Autodesk Inventor part; units mm, degrees
(part 2 of 2)
sketch "スケッチ16" plane through (0, 0, 3) normal (0, 0, 1) x (1, 0, 0)
  line L0 (-24.4121, 84.9889) -> (-12.8854, 81.652) projected
  arc A0 (-12.8854, 81.652) -> (-13.4416, 79.7309) centre (-13.1635, 80.6914) ccw projected
  line L1 (-13.4416, 79.7309) -> (-16.2223, 70.1253) projected
  arc A1 (-16.2223, 70.1253) -> (-16.7785, 68.2042) centre (-16.5004, 69.1647) ccw projected
  line L2 (-16.7785, 68.2042) -> (-28.3052, 71.5411) projected
  arc A2 (-28.3052, 71.5411) -> (-27.749, 73.4622) centre (-28.0271, 72.5017) ccw projected
  line L3 (-27.749, 73.4622) -> (-24.9683, 83.0678) projected
  arc A3 (-24.9683, 83.0678) -> (-24.4121, 84.9889) centre (-24.6902, 84.0284) ccw projected
  circle A4 centre (-11.9503, 74.0939) radius 1.5 projected
  circle A5 centre (-6.1515, 120.3493) radius 1.5 projected
  circle A6 centre (-24.1421, 119.7668) radius 1.5 projected
  circle A7 centre (-29.2403, 79.0993) radius 1.5 projected
  arc A8 (-9.3765, 127.2485) -> (-9.3118, 125.2496) centre (-9.3441, 126.249) ccw projected
  line L4 (-9.3118, 125.2496) -> (-8.9882, 115.2548) projected
  arc A9 (-8.9882, 115.2548) -> (-8.9234, 113.2558) centre (-8.9558, 114.2553) ccw projected
  line L5 (-8.9234, 113.2558) -> (-20.9172, 112.8675) projected
  arc A10 (-20.9172, 112.8675) -> (-20.9819, 114.8665) centre (-20.9495, 113.867) ccw projected
  line L6 (-20.9819, 114.8665) -> (-21.3055, 124.8612) projected
  arc A11 (-21.3055, 124.8612) -> (-21.3702, 126.8602) centre (-21.3378, 125.8607) ccw projected
  line L7 (-21.3702, 126.8602) -> (-9.3765, 127.2485) projected
  circle A12 centre (55.4, 111) radius 1.25 projected
  circle A13 centre (25, 100.25) radius 1.5 projected
  circle A14 centre (0, 66.75) radius 1.5 projected
  circle A15 centre (25, 66.75) radius 1.5 projected
  circle A16 centre (0, 100.25) radius 1.5 projected
  circle A17 centre (55.3, 64) radius 1.6 projected
  line L8 (23, 137) -> (23, 140) projected
  arc A18 (23, 140) -> (25, 140) centre (24, 140) ccw projected
  line L9 (25, 140) -> (29, 140) projected
  arc A19 (29, 140) -> (29.866, 138.5) centre (29, 139) ccw projected
  arc A20 (29.866, 138.5) -> (29, 137) centre (29, 138) ccw projected
  line L10 (29, 137) -> (25, 137) projected
  arc A21 (25, 137) -> (23, 137) centre (24, 137) ccw projected
  line L11 (51, 140) -> (55, 140) projected
  arc A22 (55, 140) -> (57, 140) centre (56, 140) ccw projected
  line L12 (57, 140) -> (57, 137) projected
  arc A23 (57, 137) -> (55, 137) centre (56, 137) ccw projected
  line L13 (55, 137) -> (51, 137) projected
  arc A24 (51, 137) -> (50.134, 138.5) centre (51, 138) ccw projected
  arc A25 (50.134, 138.5) -> (51, 140) centre (51, 139) ccw projected
  line L14 (37, 137) -> (37, 140) projected
  arc A26 (37, 140) -> (39, 140) centre (38, 140) ccw projected
  line L15 (39, 140) -> (43, 140) projected
  arc A27 (43, 140) -> (43.866, 138.5) centre (43, 139) ccw projected
  arc A28 (43.866, 138.5) -> (43, 137) centre (43, 138) ccw projected
  line L16 (43, 137) -> (39, 137) projected
  arc A29 (39, 137) -> (37, 137) centre (38, 137) ccw projected
  circle A30 centre (-12.461, 47.5151) radius 1.2295 projected
  circle A31 centre (-34.1345, 137.9496) radius 1.2295 projected
  circle A32 centre (-19.3858, 140.684) radius 1.2295 projected
  circle A33 centre (-30.5132, 56.1243) radius 1.2295 projected
  circle A34 centre (-1.5, 36) radius 1.6 projected
  circle A35 centre (-1.5, 144) radius 1.6 projected
  circle A36 centre (30, 16) radius 1.6 projected
  circle A37 centre (30, 124) radius 1.6 projected
  line L17 (62.5, 150) -> (-47.5, 150) projected
  line L18 (-47.5, 150) -> (-47.5, 10) projected
  line L19 (-47.5, 10) -> (62.5, 10) projected
  line L20 (62.5, 10) -> (62.5, 150) projected
  arc A38 (59.9998, 139.9632) -> (56.3191, 143.9873) centre (56, 140) ccw
  arc A39 (-35.0095, 55.9402) -> (-33.9034, 53.1651) centre (-30.5132, 56.1243) ccw
  arc A40 (-34.9519, 142.0993) -> (-38.3604, 137.7765) centre (-34.1345, 137.9496) ccw
  line L21 (-20.2327, 144.9986) -> (-34.9519, 142.0993)
  line L22 (-38.3604, 137.7765) -> (-35.0095, 55.9402)
  line L23 (6.5, 10) -> (30, 10)
  line L24 (59.2998, 63.9632) -> (59.9998, 139.9632)
  arc A41 (-1.133, 148.5853) -> (-2.389, 148.5133) centre (-1.5, 144) ccw
  line L25 (-20.2327, 144.9986) -> (-2.389, 148.5133)
  line L26 (-1.133, 148.5853) -> (56.3191, 143.9873)
  circle A42 centre (21.5, 22) radius 1.6 projected
  arc A43 (18.5, 15) -> (18.5, 17) centre (18.5, 16) ccw projected
  line L27 (18.5, 15) -> (6.5, 15) projected
  arc A44 (6.5, 17) -> (6.5, 15) centre (6.5, 16) ccw projected
  line L28 (6.5, 17) -> (6.5, 27) projected
  arc A45 (6.5, 29) -> (6.5, 27) centre (6.5, 28) ccw projected
  line L29 (6.5, 29) -> (18.5, 29) projected
  arc A46 (18.5, 27) -> (18.5, 29) centre (18.5, 28) ccw projected
  line L30 (18.5, 27) -> (18.5, 17) projected
  circle A47 centre (3.5, 22) radius 1.6 projected
  arc A48 (1.9797, 12.0545) -> (6.5, 10) centre (6.5, 16) ccw
  line L31 (-33.9034, 53.1651) -> (1.9797, 12.0545)
  circle A49 centre (43.2987, 57.3213) radius 1.25 projected
  circle A50 centre (43.3013, 22.6802) radius 1.25 projected
  line L32 (35.3, 23.7) -> (33.3, 23.7) projected
  line L33 (33.3, 56.3) -> (35.3, 56.3) projected
  circle A51 centre (13.3, 39.9985) radius 1.25 projected
  circle A52 centre (55.4, 87) radius 1.2295 projected
  arc A53 (45.0562, 20.5259) -> (42.136, 25.2027) centre (43.3013, 22.6802) ccw
  arc A54 (30, 10) -> (33.7894, 11.3481) centre (30, 16) ccw
  line L34 (33.7894, 11.3481) -> (45.0562, 20.5259)
  arc A55 (56.9267, 60.3457) -> (59.2998, 63.9632) centre (55.3, 64) ccw
  arc A56 (42.1337, 54.7983) -> (44.4288, 54.7825) centre (43.2987, 57.3213) ccw
  line L35 (56.9267, 60.3457) -> (44.4288, 54.7825)
  arc A57 (35.3, 23.7) -> (42.136, 25.2027) centre (35.3, 40) ccw
  arc A58 (42.1337, 54.7983) -> (35.3, 56.3) centre (35.3, 40) ccw
  arc A59 (33.3, 56.3) -> (33.3, 23.7) centre (33.3, 40) ccw
  point P0 (0, 0)
  dimension "d161" = 3
  dimension "d163" = 3
  dimension "d164" = 4
  dimension "d185" = 6
  dimension "d206" = 4
  dimension "d207" = 6
  dimension "d209" = 12
  dimension "d210" = 16.3
  dimension "d231" = 4.5
  constraints: 50 centre point, 25 point on circle, 19 tangent, 18 end point, 4 coincident, 1 collinear, 1 concentric
  measures "d161" radial gap between concentric circles of A31 A40
  measures "d163" radial gap between concentric circles of A35 A41
  measures "d164" radius of A38
  measures "d185" radius of A48
  measures "d206" distance from line of L24 A17.centre
  measures "d207" distance from line of L23 A36.centre
  measures "d209" diameter of A54
  measures "d210" radius of A57
  measures "d231" radius of A39
extrude "型抜き" cut sketch "スケッチ16" against normal through all contours A20 A19 | L8 A18 L9 A19 A20 L10 A21 | A25 A24 | L11 A22 L12 A23 L13 A24 A25 | A28 A27 | L14 A26 L15 A27 A28 L16 A29 | L19 A48 L31 A39 L22 A40 L21 L25 A41 L26 A38 L24 A55 L35 A56 A58 L33 A59 L32 A57 A53 L34 A54 | A42 | L27 A44 L28 A45 L29 A46 L30 A43 | A47 | A49 | A50 | A51 | A52 keep common part
sketch "スケッチ23" plane through (0, 0, 0) normal (0, 0, -1) x (-1, 0, 0)
  circle A0 centre (-30, 124) radius 1.6 projected
  circle A1 centre (-30, 16) radius 1.6 projected
  circle A2 centre (1.5, 144) radius 1.6 projected
  circle A3 centre (1.5, 36) radius 1.6 projected
  circle A4 centre (30.5132, 56.1243) radius 1.2295 projected
  circle A5 centre (19.3858, 140.684) radius 1.2295 projected
  circle A6 centre (34.1345, 137.9496) radius 1.2295 projected
  circle A7 centre (12.461, 47.5151) radius 1.2295 projected
  line L0 (-37, 140) -> (-37, 137) projected
  arc A8 (-39, 137) -> (-37, 137) centre (-38, 137) ccw projected
  line L1 (-39, 137) -> (-43, 137) projected
  arc A9 (-43.866, 138.5) -> (-43, 137) centre (-43, 138) ccw projected
  arc A10 (-43, 140) -> (-43.866, 138.5) centre (-43, 139) ccw projected
  line L2 (-43, 140) -> (-39, 140) projected
  arc A11 (-37, 140) -> (-39, 140) centre (-38, 140) ccw projected
  line L3 (-55, 140) -> (-51, 140) projected
  arc A12 (-50.134, 138.5) -> (-51, 140) centre (-51, 139) ccw projected
  arc A13 (-51, 137) -> (-50.134, 138.5) centre (-51, 138) ccw projected
  line L4 (-51, 137) -> (-55, 137) projected
  arc A14 (-57, 137) -> (-55, 137) centre (-56, 137) ccw projected
  line L5 (-57, 137) -> (-57, 140) projected
  arc A15 (-55, 140) -> (-57, 140) centre (-56, 140) ccw projected
  line L6 (-23, 140) -> (-23, 137) projected
  arc A16 (-25, 137) -> (-23, 137) centre (-24, 137) ccw projected
  line L7 (-25, 137) -> (-29, 137) projected
  arc A17 (-29.866, 138.5) -> (-29, 137) centre (-29, 138) ccw projected
  arc A18 (-29, 140) -> (-29.866, 138.5) centre (-29, 139) ccw projected
  line L8 (-29, 140) -> (-25, 140) projected
  arc A19 (-23, 140) -> (-25, 140) centre (-24, 140) ccw projected
  circle A20 centre (-55.3, 64) radius 1.6 projected
  circle A21 centre (0, 100.25) radius 1.5 projected
  circle A22 centre (-25, 66.75) radius 1.5 projected
  circle A23 centre (0, 66.75) radius 1.5 projected
  circle A24 centre (-25, 100.25) radius 1.5 projected
  circle A25 centre (-55.4, 87) radius 1.25 projected
  circle A26 centre (-55.4, 111) radius 1.25 projected
  arc A27 (9.3765, 127.2485) -> (9.3118, 125.2496) centre (9.3441, 126.249) ccw projected
  line L9 (9.3765, 127.2485) -> (21.3702, 126.8602) projected
  arc A28 (21.3055, 124.8612) -> (21.3702, 126.8602) centre (21.3378, 125.8607) ccw projected
  line L10 (21.3055, 124.8612) -> (20.9819, 114.8665) projected
  arc A29 (20.9172, 112.8675) -> (20.9819, 114.8665) centre (20.9495, 113.867) ccw projected
  line L11 (20.9172, 112.8675) -> (8.9234, 113.2558) projected
  arc A30 (8.9882, 115.2548) -> (8.9234, 113.2558) centre (8.9558, 114.2553) ccw projected
  line L12 (8.9882, 115.2548) -> (9.3118, 125.2496) projected
  circle A31 centre (29.2403, 79.0993) radius 1.5 projected
  circle A32 centre (24.1421, 119.7668) radius 1.5 projected
  circle A33 centre (6.1515, 120.3493) radius 1.5 projected
  circle A34 centre (11.9503, 74.0939) radius 1.5 projected
  line L13 (12.8854, 81.652) -> (24.4121, 84.9889) projected
  arc A35 (24.9683, 83.0678) -> (24.4121, 84.9889) centre (24.6902, 84.0284) ccw projected
  line L14 (24.9683, 83.0678) -> (27.749, 73.4622) projected
  arc A36 (28.3052, 71.5411) -> (27.749, 73.4622) centre (28.0271, 72.5017) ccw projected
  line L15 (28.3052, 71.5411) -> (16.7785, 68.2042) projected
  arc A37 (16.2223, 70.1253) -> (16.7785, 68.2042) centre (16.5004, 69.1647) ccw projected
  line L16 (16.2223, 70.1253) -> (13.4416, 79.7309) projected
  arc A38 (12.8854, 81.652) -> (13.4416, 79.7309) centre (13.1635, 80.6914) ccw projected
  circle A39 centre (-21.5, 22) radius 1.6 projected
  circle A40 centre (-21.5, 124) radius 1.6 projected
  arc A41 (-6.5, 129) -> (-6.5, 131) centre (-6.5, 130) ccw projected
  line L17 (-6.5, 129) -> (-6.5, 119) projected
  arc A42 (-6.5, 117) -> (-6.5, 119) centre (-6.5, 118) ccw projected
  line L18 (-6.5, 117) -> (-18.5, 117) projected
  arc A43 (-18.5, 119) -> (-18.5, 117) centre (-18.5, 118) ccw projected
  line L19 (-18.5, 119) -> (-18.5, 129) projected
  arc A44 (-18.5, 131) -> (-18.5, 129) centre (-18.5, 130) ccw projected
  line L20 (-18.5, 131) -> (-6.5, 131) projected
  arc A45 (-18.5, 17) -> (-18.5, 15) centre (-18.5, 16) ccw projected
  line L21 (-18.5, 17) -> (-18.5, 27) projected
  arc A46 (-18.5, 29) -> (-18.5, 27) centre (-18.5, 28) ccw projected
  line L22 (-18.5, 29) -> (-6.5, 29) projected
  arc A47 (-6.5, 27) -> (-6.5, 29) centre (-6.5, 28) ccw projected
  line L23 (-6.5, 27) -> (-6.5, 17) projected
  arc A48 (-6.5, 15) -> (-6.5, 17) centre (-6.5, 16) ccw projected
  line L24 (-6.5, 15) -> (-18.5, 15) projected
  circle A49 centre (-3.5, 124) radius 1.6 projected
  circle A50 centre (-3.5, 22) radius 1.6 projected
  circle A51 centre (-43.3013, 22.6802) radius 1.25 projected
  circle A52 centre (-13.3, 39.9985) radius 1.25 projected
  circle A53 centre (-43.2987, 57.3213) radius 1.25 projected
  arc A54 (-42.136, 25.2027) -> (-45.0562, 20.5259) centre (-43.3013, 22.6802) ccw projected
  line L25 (-33.7894, 11.3481) -> (-45.0562, 20.5259) projected
  arc A55 (-33.7894, 11.3481) -> (-30, 10) centre (-30, 16) ccw projected
  line L26 (-30, 10) -> (-6.5, 10) projected
  arc A56 (-6.5, 10) -> (-1.9797, 12.0545) centre (-6.5, 16) ccw projected
  line L27 (33.9034, 53.1651) -> (-1.9797, 12.0545) projected
  arc A57 (33.9034, 53.1651) -> (35.0095, 55.9402) centre (30.5132, 56.1243) ccw projected
  line L28 (38.3604, 137.7765) -> (35.0095, 55.9402) projected
  arc A58 (38.3604, 137.7765) -> (34.9519, 142.0993) centre (34.1345, 137.9496) ccw projected
  line L29 (2.389, 148.5133) -> (34.9519, 142.0993) projected
  arc A59 (2.389, 148.5133) -> (1.133, 148.5853) centre (1.5, 144) ccw projected
  line L30 (-56.3191, 143.9873) -> (1.133, 148.5853) projected
  arc A60 (-56.3191, 143.9873) -> (-59.9998, 139.9632) centre (-56, 140) ccw projected
  line L31 (-59.2998, 63.9632) -> (-59.9998, 139.9632) projected
  arc A61 (-59.2998, 63.9632) -> (-56.9267, 60.3457) centre (-55.3, 64) ccw projected
  line L32 (-44.4288, 54.7825) -> (-56.9267, 60.3457) projected
  arc A62 (-44.4288, 54.7825) -> (-42.1337, 54.7983) centre (-43.2987, 57.3213) ccw projected
  arc A63 (-35.3, 56.3) -> (-42.1337, 54.7983) centre (-35.3, 40) ccw projected
  line L33 (-35.3, 56.3) -> (-33.3, 56.3) projected
  arc A64 (-33.3, 23.7) -> (-33.3, 56.3) centre (-33.3, 40) ccw projected
  line L34 (-33.3, 23.7) -> (-35.3, 23.7) projected
  arc A65 (-42.136, 25.2027) -> (-35.3, 23.7) centre (-35.3, 40) ccw projected
  circle A66 centre (-35, 83.5) radius 1.2295 projected
  circle A67 centre (-45, 98.5) radius 1.2295 projected
  circle A68 centre (-45, 68.5) radius 1.2295 projected
  arc A69 (4.5938, 147.4041) -> (1.133, 148.5853) centre (1.5, 144) ccw
  arc A70 (33.9034, 53.1651) -> (34.9806, 56.6656) centre (30.5132, 56.1243) ccw
  arc A71 (32.2185, 79.4601) -> (32.217, 79.4724) centre (29.2403, 79.0993) ccw
  arc A72 (27.1188, 120.1399) -> (26.8457, 121.067) centre (24.1421, 119.7668) ccw
  line L35 (21.3702, 126.8602) -> (21.5321, 131.8602) construction
  line L36 (21.5321, 131.8602) -> (18.5321, 131.9573) construction
  arc A73 (22.1292, 130.8741) -> (20.7575, 132.7138) centre (16.722, 128.2737) ccw
  line L37 (20.7575, 132.7138) -> (4.5938, 147.4041)
  line L38 (22.1292, 130.8741) -> (26.8457, 121.067)
  line L39 (27.1188, 120.1399) -> (32.217, 79.4724)
  line L40 (32.2185, 79.4601) -> (34.9806, 56.6656)
  point P0 (0, 0)
  dimension "d233" = 6
  dimension "d234" = 6
  dimension "d235" = 5
  dimension "d236" = 3
  dimension "d237" = 6
  constraints: 14 end point, 11 point on circle, 8 tangent, 5 centre point, 3 coincident, 2 perpendicular
  measures "d233" diameter of A71
  measures "d234" diameter of A72
  measures "d235" vertical distance of L35.end L9.end
  measures "d236" horizontal distance of L35.end L36.end
  measures "d237" radius of A73
extrude "押し出し17" cut sketch "スケッチ23" against normal through all contours A70 L40 A71 L39 A72 L38 A73 L37 A69 L29 A58 L28
sketch "スケッチ24" plane through (0, 0, 0) normal (0, 0, -1) x (-1, 0, 0)
  circle A0 centre (-45, 68.5) radius 1.2295 projected
  circle A1 centre (-45, 98.5) radius 1.2295 projected
  circle A2 centre (-35, 83.5) radius 1.2295 projected
  arc A3 (33.9034, 53.1651) -> (34.9806, 56.6656) centre (30.5132, 56.1243) ccw projected
  line L0 (34.9806, 56.6656) -> (32.2185, 79.4601) projected
  arc A4 (32.2185, 79.4601) -> (32.217, 79.4724) centre (29.2403, 79.0993) ccw projected
  line L1 (32.217, 79.4724) -> (27.1188, 120.1399) projected
  arc A5 (27.1188, 120.1399) -> (26.8457, 121.067) centre (24.1421, 119.7668) ccw projected
  line L2 (26.8457, 121.067) -> (22.1292, 130.8741) projected
  arc A6 (22.1292, 130.8741) -> (20.7575, 132.7138) centre (16.722, 128.2737) ccw projected
  line L3 (20.7575, 132.7138) -> (4.5938, 147.4041) projected
  arc A7 (4.5938, 147.4041) -> (1.133, 148.5853) centre (1.5, 144) ccw projected
  line L4 (-56.3191, 143.9873) -> (1.133, 148.5853) projected
  arc A8 (-56.3191, 143.9873) -> (-59.9998, 139.9632) centre (-56, 140) ccw projected
  line L5 (-59.2998, 63.9632) -> (-59.9998, 139.9632) projected
  arc A9 (-59.2998, 63.9632) -> (-56.9267, 60.3457) centre (-55.3, 64) ccw projected
  line L6 (-44.4288, 54.7825) -> (-56.9267, 60.3457) projected
  arc A10 (-44.4288, 54.7825) -> (-42.1337, 54.7983) centre (-43.2987, 57.3213) ccw projected
  arc A11 (-35.3, 56.3) -> (-42.1337, 54.7983) centre (-35.3, 40) ccw projected
  line L7 (-35.3, 56.3) -> (-33.3, 56.3) projected
  arc A12 (-33.3, 23.7) -> (-33.3, 56.3) centre (-33.3, 40) ccw projected
  line L8 (-33.3, 23.7) -> (-35.3, 23.7) projected
  arc A13 (-42.136, 25.2027) -> (-35.3, 23.7) centre (-35.3, 40) ccw projected
  arc A14 (-42.136, 25.2027) -> (-45.0562, 20.5259) centre (-43.3013, 22.6802) ccw projected
  line L9 (-33.7894, 11.3481) -> (-45.0562, 20.5259) projected
  arc A15 (-33.7894, 11.3481) -> (-30, 10) centre (-30, 16) ccw projected
  line L10 (-30, 10) -> (-6.5, 10) projected
  arc A16 (-6.5, 10) -> (-1.9797, 12.0545) centre (-6.5, 16) ccw projected
  line L11 (33.9034, 53.1651) -> (-1.9797, 12.0545) projected
  circle A17 centre (-43.2987, 57.3213) radius 1.25 projected
  circle A18 centre (-13.3, 39.9985) radius 1.25 projected
  circle A19 centre (-43.3013, 22.6802) radius 1.25 projected
  circle A20 centre (-3.5, 22) radius 1.6 projected
  circle A21 centre (-3.5, 124) radius 1.6 projected
  arc A22 (-18.5, 17) -> (-18.5, 15) centre (-18.5, 16) ccw projected
  line L12 (-18.5, 17) -> (-18.5, 27) projected
  arc A23 (-18.5, 29) -> (-18.5, 27) centre (-18.5, 28) ccw projected
  line L13 (-18.5, 29) -> (-6.5, 29) projected
  arc A24 (-6.5, 27) -> (-6.5, 29) centre (-6.5, 28) ccw projected
  line L14 (-6.5, 27) -> (-6.5, 17) projected
  arc A25 (-6.5, 15) -> (-6.5, 17) centre (-6.5, 16) ccw projected
  line L15 (-6.5, 15) -> (-18.5, 15) projected
  arc A26 (-6.5, 129) -> (-6.5, 131) centre (-6.5, 130) ccw projected
  line L16 (-6.5, 129) -> (-6.5, 119) projected
  arc A27 (-6.5, 117) -> (-6.5, 119) centre (-6.5, 118) ccw projected
  line L17 (-6.5, 117) -> (-18.5, 117) projected
  arc A28 (-18.5, 119) -> (-18.5, 117) centre (-18.5, 118) ccw projected
  line L18 (-18.5, 119) -> (-18.5, 129) projected
  arc A29 (-18.5, 131) -> (-18.5, 129) centre (-18.5, 130) ccw projected
  line L19 (-18.5, 131) -> (-6.5, 131) projected
  circle A30 centre (-21.5, 124) radius 1.6 projected
  circle A31 centre (-21.5, 22) radius 1.6 projected
  line L20 (12.8854, 81.652) -> (24.4121, 84.9889) projected
  arc A32 (24.9683, 83.0678) -> (24.4121, 84.9889) centre (24.6902, 84.0284) ccw projected
  line L21 (24.9683, 83.0678) -> (27.749, 73.4622) projected
  arc A33 (28.3052, 71.5411) -> (27.749, 73.4622) centre (28.0271, 72.5017) ccw projected
  line L22 (28.3052, 71.5411) -> (16.7785, 68.2042) projected
  arc A34 (16.2223, 70.1253) -> (16.7785, 68.2042) centre (16.5004, 69.1647) ccw projected
  line L23 (16.2223, 70.1253) -> (13.4416, 79.7309) projected
  arc A35 (12.8854, 81.652) -> (13.4416, 79.7309) centre (13.1635, 80.6914) ccw projected
  circle A36 centre (11.9503, 74.0939) radius 1.5 projected
  circle A37 centre (6.1515, 120.3493) radius 1.5 projected
  circle A38 centre (24.1421, 119.7668) radius 1.5 projected
  circle A39 centre (29.2403, 79.0993) radius 1.5 projected
  arc A40 (9.3765, 127.2485) -> (9.3118, 125.2496) centre (9.3441, 126.249) ccw projected
  line L24 (9.3765, 127.2485) -> (21.3702, 126.8602) projected
  arc A41 (21.3055, 124.8612) -> (21.3702, 126.8602) centre (21.3378, 125.8607) ccw projected
  line L25 (21.3055, 124.8612) -> (20.9819, 114.8665) projected
  arc A42 (20.9172, 112.8675) -> (20.9819, 114.8665) centre (20.9495, 113.867) ccw projected
  line L26 (20.9172, 112.8675) -> (8.9234, 113.2558) projected
  arc A43 (8.9882, 115.2548) -> (8.9234, 113.2558) centre (8.9558, 114.2553) ccw projected
  line L27 (8.9882, 115.2548) -> (9.3118, 125.2496) projected
  circle A44 centre (-55.4, 111) radius 1.25 projected
  circle A45 centre (-55.4, 87) radius 1.25 projected
  circle A46 centre (-25, 100.25) radius 1.5 projected
  circle A47 centre (0, 66.75) radius 1.5 projected
  circle A48 centre (-25, 66.75) radius 1.5 projected
  circle A49 centre (0, 100.25) radius 1.5 projected
  circle A50 centre (-55.3, 64) radius 1.6 projected
  line L28 (-23, 140) -> (-23, 137) projected
  arc A51 (-25, 137) -> (-23, 137) centre (-24, 137) ccw projected
  line L29 (-25, 137) -> (-29, 137) projected
  arc A52 (-29.866, 138.5) -> (-29, 137) centre (-29, 138) ccw projected
  arc A53 (-29, 140) -> (-29.866, 138.5) centre (-29, 139) ccw projected
  line L30 (-29, 140) -> (-25, 140) projected
  arc A54 (-23, 140) -> (-25, 140) centre (-24, 140) ccw projected
  line L31 (-55, 140) -> (-51, 140) projected
  arc A55 (-50.134, 138.5) -> (-51, 140) centre (-51, 139) ccw projected
  arc A56 (-51, 137) -> (-50.134, 138.5) centre (-51, 138) ccw projected
  line L32 (-51, 137) -> (-55, 137) projected
  arc A57 (-57, 137) -> (-55, 137) centre (-56, 137) ccw projected
  line L33 (-57, 137) -> (-57, 140) projected
  arc A58 (-55, 140) -> (-57, 140) centre (-56, 140) ccw projected
  line L34 (-37, 140) -> (-37, 137) projected
  arc A59 (-39, 137) -> (-37, 137) centre (-38, 137) ccw projected
  line L35 (-39, 137) -> (-43, 137) projected
  arc A60 (-43.866, 138.5) -> (-43, 137) centre (-43, 138) ccw projected
  arc A61 (-43, 140) -> (-43.866, 138.5) centre (-43, 139) ccw projected
  line L36 (-43, 140) -> (-39, 140) projected
  arc A62 (-37, 140) -> (-39, 140) centre (-38, 140) ccw projected
  circle A63 centre (12.461, 47.5151) radius 1.2295 projected
  circle A64 centre (30.5132, 56.1243) radius 1.2295 projected
  circle A65 centre (1.5, 36) radius 1.6 projected
  circle A66 centre (1.5, 144) radius 1.6 projected
  circle A67 centre (-30, 16) radius 1.6 projected
  circle A68 centre (-30, 124) radius 1.6 projected
  line L37 (107.7557, 84.6522) -> (35.5469, 50.2156) projected
  line L38 (35.5469, 50.2156) -> (36.8383, 47.5078) projected
  line L39 (109.0471, 81.9444) -> (36.8383, 47.5078) projected
  line L40 (107.7557, 84.6522) -> (109.0471, 81.9444) projected
  line L41 (95.9872, 80.6171) -> (4.2149, 147.7134)
  arc A69 (4.5938, 147.4041) -> (1.133, 148.5853) centre (1.5, 144) ccw projected
  line L42 (34.6916, 49.6035) -> (-2.2067, 11.8086)
  arc A70 (96.9244, 79.4867) -> (95.9872, 80.6171) centre (94.2166, 78.1954) ccw
  arc A71 (35.5469, 50.2156) -> (34.6916, 49.6035) centre (36.8383, 47.5078) ccw
  point P0 (0, 0)
  dimension "d244" = 15
  dimension "d245" = 3
  constraints: 6 point on circle, 5 tangent, 4 end point, 2 centre point, 1 equal radius, 1 line through centre, 1 point on line
  measures "d244" distance from line of L40 A70.centre
  measures "d245" radius of A70
extrude "押し出し18" add sketch "スケッチ24" against normal blind 3 contours A3 L0 A4 L1 A5 L2 A6 L3 A7 L41 A70 L37 A71 L42 A16 L11
sketch "スケッチ25" plane through (0, 0, 0) normal (0, 0, -1) x (-1, 0, 0)
  circle A0 centre (-45, 68.5) radius 1.2295 projected
  circle A1 centre (-45, 98.5) radius 1.2295 projected
  circle A2 centre (-35, 83.5) radius 1.2295 projected
  line L0 (-2.2067, 11.8086) -> (34.6916, 49.6035) projected
  arc A3 (34.6916, 49.6035) -> (35.5469, 50.2156) centre (36.8383, 47.5078) ccw projected
  line L1 (35.5469, 50.2156) -> (96.9244, 79.4867)
  arc A4 (96.9244, 79.4867) -> (95.9872, 80.6171) centre (94.2166, 78.1954) ccw projected
  line L2 (95.9872, 80.6171) -> (4.2149, 147.7134) projected
  arc A5 (1.133, 148.5853) -> (4.2149, 147.7134) centre (1.5, 144) ccw projected
  line L3 (-56.3191, 143.9873) -> (1.133, 148.5853) projected
  arc A6 (-59.9998, 139.9632) -> (-56.3191, 143.9873) centre (-56, 140) ccw projected
  line L4 (-59.2998, 63.9632) -> (-59.9998, 139.9632) projected
  arc A7 (-56.9267, 60.3457) -> (-59.2998, 63.9632) centre (-55.3, 64) ccw projected
  line L5 (-44.4288, 54.7825) -> (-56.9267, 60.3457) projected
  arc A8 (-42.1337, 54.7983) -> (-44.4288, 54.7825) centre (-43.2987, 57.3213) ccw projected
  arc A9 (-42.1337, 54.7983) -> (-35.3, 56.3) centre (-35.3, 40) ccw projected
  line L6 (-35.3, 56.3) -> (-33.3, 56.3) projected
  arc A10 (-33.3, 56.3) -> (-33.3, 23.7) centre (-33.3, 40) ccw projected
  line L7 (-33.3, 23.7) -> (-35.3, 23.7) projected
  arc A11 (-35.3, 23.7) -> (-42.136, 25.2027) centre (-35.3, 40) ccw projected
  arc A12 (-45.0562, 20.5259) -> (-42.136, 25.2027) centre (-43.3013, 22.6802) ccw projected
  line L8 (-33.7894, 11.3481) -> (-45.0562, 20.5259) projected
  arc A13 (-30, 10) -> (-33.7894, 11.3481) centre (-30, 16) ccw projected
  line L9 (-30, 10) -> (-6.5, 10) projected
  arc A14 (-2.2067, 11.8086) -> (-6.5, 10) centre (-6.5, 16) ccw projected
  circle A15 centre (-43.2987, 57.3213) radius 1.25 projected
  circle A16 centre (-13.3, 39.9985) radius 1.25 projected
  circle A17 centre (-43.3013, 22.6802) radius 1.25 projected
  circle A18 centre (-3.5, 22) radius 1.6 projected
  circle A19 centre (-3.5, 124) radius 1.6 projected
  arc A20 (-18.5, 15) -> (-18.5, 17) centre (-18.5, 16) ccw projected
  line L10 (-18.5, 17) -> (-18.5, 27) projected
  arc A21 (-18.5, 27) -> (-18.5, 29) centre (-18.5, 28) ccw projected
  line L11 (-18.5, 29) -> (-6.5, 29) projected
  arc A22 (-6.5, 29) -> (-6.5, 27) centre (-6.5, 28) ccw projected
  line L12 (-6.5, 27) -> (-6.5, 17) projected
  arc A23 (-6.5, 17) -> (-6.5, 15) centre (-6.5, 16) ccw projected
  line L13 (-6.5, 15) -> (-18.5, 15) projected
  arc A24 (-6.5, 131) -> (-6.5, 129) centre (-6.5, 130) ccw projected
  line L14 (-6.5, 129) -> (-6.5, 119) projected
  arc A25 (-6.5, 119) -> (-6.5, 117) centre (-6.5, 118) ccw projected
  line L15 (-6.5, 117) -> (-18.5, 117) projected
  arc A26 (-18.5, 117) -> (-18.5, 119) centre (-18.5, 118) ccw projected
  line L16 (-18.5, 119) -> (-18.5, 129) projected
  arc A27 (-18.5, 129) -> (-18.5, 131) centre (-18.5, 130) ccw projected
  line L17 (-18.5, 131) -> (-6.5, 131) projected
  circle A28 centre (-21.5, 124) radius 1.6 projected
  circle A29 centre (-21.5, 22) radius 1.6 projected
  line L18 (12.8854, 81.652) -> (24.4121, 84.9889) projected
  arc A30 (24.4121, 84.9889) -> (24.9683, 83.0678) centre (24.6902, 84.0284) ccw projected
  line L19 (24.9683, 83.0678) -> (27.749, 73.4622) projected
  arc A31 (27.749, 73.4622) -> (28.3052, 71.5411) centre (28.0271, 72.5017) ccw projected
  line L20 (28.3052, 71.5411) -> (16.7785, 68.2042) projected
  arc A32 (16.7785, 68.2042) -> (16.2223, 70.1253) centre (16.5004, 69.1647) ccw projected
  line L21 (16.2223, 70.1253) -> (13.4416, 79.7309) projected
  arc A33 (13.4416, 79.7309) -> (12.8854, 81.652) centre (13.1635, 80.6914) ccw projected
  circle A34 centre (11.9503, 74.0939) radius 1.5 projected
  circle A35 centre (6.1515, 120.3493) radius 1.5 projected
  circle A36 centre (24.1421, 119.7668) radius 1.5 projected
  circle A37 centre (29.2403, 79.0993) radius 1.5 projected
  arc A38 (9.3118, 125.2496) -> (9.3765, 127.2485) centre (9.3441, 126.249) ccw projected
  line L22 (9.3765, 127.2485) -> (21.3702, 126.8602) projected
  arc A39 (21.3702, 126.8602) -> (21.3055, 124.8612) centre (21.3378, 125.8607) ccw projected
  line L23 (21.3055, 124.8612) -> (20.9819, 114.8665) projected
  arc A40 (20.9819, 114.8665) -> (20.9172, 112.8675) centre (20.9495, 113.867) ccw projected
  line L24 (20.9172, 112.8675) -> (8.9234, 113.2558) projected
  arc A41 (8.9234, 113.2558) -> (8.9882, 115.2548) centre (8.9558, 114.2553) ccw projected
  line L25 (8.9882, 115.2548) -> (9.3118, 125.2496) projected
  circle A42 centre (-55.4, 111) radius 1.25 projected
  circle A43 centre (-55.4, 87) radius 1.25 projected
  circle A44 centre (-25, 100.25) radius 1.5 projected
  circle A45 centre (0, 66.75) radius 1.5 projected
  circle A46 centre (-25, 66.75) radius 1.5 projected
  circle A47 centre (0, 100.25) radius 1.5 projected
  circle A48 centre (-55.3, 64) radius 1.6 projected
  line L26 (-23, 140) -> (-23, 137) projected
  arc A49 (-23, 137) -> (-25, 137) centre (-24, 137) ccw projected
  line L27 (-25, 137) -> (-29, 137) projected
  arc A50 (-29, 137) -> (-29.866, 138.5) centre (-29, 138) ccw projected
  arc A51 (-29.866, 138.5) -> (-29, 140) centre (-29, 139) ccw projected
  line L28 (-29, 140) -> (-25, 140) projected
  arc A52 (-25, 140) -> (-23, 140) centre (-24, 140) ccw projected
  line L29 (-55, 140) -> (-51, 140) projected
  arc A53 (-51, 140) -> (-50.134, 138.5) centre (-51, 139) ccw projected
  arc A54 (-50.134, 138.5) -> (-51, 137) centre (-51, 138) ccw projected
  line L30 (-51, 137) -> (-55, 137) projected
  arc A55 (-55, 137) -> (-57, 137) centre (-56, 137) ccw projected
  line L31 (-57, 137) -> (-57, 140) projected
  arc A56 (-57, 140) -> (-55, 140) centre (-56, 140) ccw projected
  line L32 (-37, 140) -> (-37, 137) projected
  arc A57 (-37, 137) -> (-39, 137) centre (-38, 137) ccw projected
  line L33 (-39, 137) -> (-43, 137) projected
  arc A58 (-43, 137) -> (-43.866, 138.5) centre (-43, 138) ccw projected
  arc A59 (-43.866, 138.5) -> (-43, 140) centre (-43, 139) ccw projected
  line L34 (-43, 140) -> (-39, 140) projected
  arc A60 (-39, 140) -> (-37, 140) centre (-38, 140) ccw projected
  circle A61 centre (12.461, 47.5151) radius 1.2295 projected
  circle A62 centre (30.5132, 56.1243) radius 1.2295 projected
  circle A63 centre (1.5, 36) radius 1.6 projected
  circle A64 centre (1.5, 144) radius 1.6 projected
  circle A65 centre (-30, 16) radius 1.6 projected
  circle A66 centre (-30, 124) radius 1.6 projected
  arc A67 (93.314, 77.7649) -> (90.6061, 76.4735) centre (91.96, 77.1192) ccw
  arc A68 (72.5539, 67.8644) -> (69.8461, 66.573) centre (71.2, 67.2187) ccw
  arc A69 (62.6252, 63.1293) -> (59.9174, 61.838) centre (61.2713, 62.4837) ccw
  arc A70 (41.8652, 53.2288) -> (39.1573, 51.9374) centre (40.5112, 52.5831) ccw
  line L35 (90.6061, 76.4735) -> (94.4803, 68.35)
  line L36 (94.4803, 68.35) -> (76.428, 59.7409)
  line L37 (76.428, 59.7409) -> (72.5539, 67.8644)
  line L38 (59.9174, 61.838) -> (63.7915, 53.7145)
  line L39 (63.7915, 53.7145) -> (45.7393, 45.1053)
  line L40 (45.7393, 45.1053) -> (41.8652, 53.2288)
  line L41 (86.2034, 69.4437) -> (80.7877, 66.861) construction
  line L42 (85.5362, 70.8428) -> (80.1205, 68.26)
  line L43 (81.4549, 65.4619) -> (86.8706, 68.0447)
  arc A71 (86.8706, 68.0447) -> (85.5362, 70.8428) centre (86.2034, 69.4437) ccw
  arc A72 (80.1205, 68.26) -> (81.4549, 65.4619) centre (80.7877, 66.861) ccw
  line L44 (55.5146, 54.8081) -> (50.099, 52.2254) construction
  line L45 (54.8474, 56.2072) -> (49.4318, 53.6244)
  line L46 (50.7662, 50.8263) -> (56.1818, 53.4091)
  arc A73 (56.1818, 53.4091) -> (54.8474, 56.2072) centre (55.5146, 54.8081) ccw
  arc A74 (49.4318, 53.6244) -> (50.7662, 50.8263) centre (50.099, 52.2254) ccw
  line L47 (35.5469, 50.2156) -> (96.9244, 79.4867) projected
  line L48 (83.4956, 68.1523) -> (85.4541, 64.0455) construction
  line L49 (52.8068, 53.5168) -> (54.7654, 49.4099) construction
  circle A75 centre (47.7402, 110.9362) radius 1.6
  line L50 (47.7402, 110.9362) -> (50.101, 114.1653) construction
  circle A76 centre (78.3516, 78.9385) radius 1.25
  circle A77 centre (47.6628, 64.303) radius 1.25
  point P0 (0, 0)
  dimension "d246" = 3
  dimension "d247" = 3
  dimension "d248" = 3
  dimension "d249" = 3
  dimension "d250" = 9
  dimension "d251" = 20
  dimension "d252" = 4
  dimension "d253" = 14
  dimension "d255" = 3.1
  dimension "d256" = 6
  dimension "d261" = 3.2
  dimension "d262" = 4
  dimension "d263" = 3
  dimension "d264" = 2.5
  dimension "d265" = 2.5
  dimension "d266" = 7.5
  dimension "d267" = 7.5
  constraints: 78 centre point, 34 end point, 16 point on circle, 9 tangent, 6 perpendicular, 5 midpoint, 5 parallel, 4 collinear, 2 point on line, 1 equal radius, 17 other
  measures "d246" diameter of A67
  measures "d247" diameter of A68
  measures "d248" diameter of A69
  measures "d249" diameter of A70
  measures "d251" distance of L35.end L36.end
  measures "d252" distance of A4.start A67.start
  measures "d253" distance between parallel lines of L38 L37
  measures "d255" diameter of A74
  measures "d256" distance of L41.start L41.end
  measures "d261" diameter of A75
  measures "d262" distance from line of L2 L50.start
  measures "d263" distance between parallel lines of L43 L36
  measures "d264" diameter of A76
  measures "d265" diameter of A77
extrude "押し出し19" add sketch "スケッチ25" against normal blind 3 contours L1 L38 L39 L40 | L1 L35 L36 L37 | A71 L43 A72 L42 | A73 L46 A74 L45
extrude "押し出し20" cut sketch "スケッチ25" against normal blind 3 contours A70 L1 | A69 L1 | A68 L1 | A67 L1 | A71 L43 A72 L42 | A73 L46 A74 L45 | A75 | A76 | A77
equation "\"d2\" = d3"
equation "\"d5\" = d2"
equation "\"d8\" = d7"
